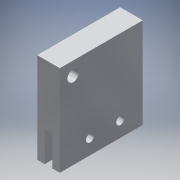
# Autodesk Inventor part: NarrowSupportForLift
Saved by Autodesk Inventor 2016 SP1 (Build 200210100, 210)
## iProperties
Created: 2016-02-14
Part Number: NarrowSupportForLift
Material: Aluminum 6061
Document SubType Name: Modeling
Designer: steele
Density: 2.7 g/cm^3
Appearance: Aluminum - Flat
Mass: 237.224 g
Surface Area: 201.153 cm^2
Volume: 87.8608 cm^3
Author: steele
Autodesk Inventor part; units mm, degrees
ref_plane "YZ Plane" through (0, 0, 0) normal (1, 0, 0) x (0, 1, 0)
ref_plane "XZ Plane" through (0, 0, 0) normal (0, 1, 0) x (-1, 0, 0)
ref_plane "XY Plane" through (0, 0, 0) normal (0, 0, 1) x (1, 0, 0)
sketch "Sketch4" plane through (0, 0, 0) normal (1, 0, 0) x (0, 1, 0)
  line L0 (-25.4, 34.925) -> (-25.4, -34.925)
  line L1 (-25.4, -34.925) -> (0, -34.925)
  line L2 (0, -34.925) -> (0, 34.925)
  line L3 (0, 34.925) -> (-25.4, 34.925)
  line L4 (-25.4, -34.925) -> (-12.7, 0) construction
  line L5 (0, 34.925) -> (50.8, 34.925)
  line L6 (50.8, 34.925) -> (50.8, -34.925)
  line L7 (50.8, -34.925) -> (0, -34.925)
  line L8 (0, -34.925) -> (0, 34.925)
  circle A0 centre (39.6875, 23.8125) radius 4.7625
  circle A1 centre (39.6875, -23.8125) radius 4.7625
  point P0 (0, 0)
  point P1 (-12.7, 0)
  dimension "d2" = 69.85
  dimension "d3" = 25.4
  dimension "d12" = 50.8
  dimension "d15" = 9.525
  dimension "d16" = 11.1125
  dimension "d23" = 11.1125
  dimension "d26" = 11.1125
  constraints: 18 end point, 4 parallel, 2 centre point, 2 perpendicular, 1 collinear, 1 equal radius, 1 horizontal, 1 point on line, 1 vertical
  measures "d2" distance of L0.start L0.end
  measures "d3" distance of L2.end L0.start
  measures "d12" distance of L2.end L5.end
  measures "d15" diameter of A0
  measures "d16" distance from line of A0.centre L6
  measures "d23" distance from line of A0.centre L5
  measures "d26" distance from line of A1.centre L7
extrude "Extrusion3" add sketch "Sketch4" along normal mid plane 19.05 contours L3 L2 L1 L0 | L5 L6 L7 L2 | A1
sketch "Sketch6" plane through (-9.525, -25.4, 34.925) normal (0, 0, 1) x (1, 0, 0)
  line L0 (9.525, 25.4) -> (9.525, 0) construction
  line L1 (0, 0) -> (19.05, 0) construction
  line L2 (6.35, 0) -> (12.7, 0)
  line L3 (12.7, 0) -> (12.7, 25.4)
  line L4 (12.7, 25.4) -> (6.35, 25.4)
  line L5 (6.35, 25.4) -> (6.35, 0)
  line L6 (6.35, 0) -> (12.7, 25.4) construction
  line L7 (12.7, 0) -> (6.35, 25.4) construction
  point P0 (9.525, 12.7)
  dimension "d20" = 6.35
  constraints: 14 end point, 4 midpoint, 2 parallel, 1 horizontal, 1 perpendicular
  measures "d20" distance between parallel lines of L3 L5
extrude "Extrusion4" cut sketch "Sketch6" against normal through all
sketch "Sketch7" plane through (9.525, 0, 0) normal (1, 0, 0) x (0, 0, -1)
  line L0 (34.925, -25.4) -> (34.925, 0) projected
  line L1 (-34.925, -25.4) -> (34.925, -25.4) projected
  line L2 (-34.925, 0) -> (-34.925, -25.4) projected
  line L3 (-34.925, 0) -> (34.925, 0) projected
  line L4 (-34.925, -85.725) -> (-34.925, -12.7) projected
  arc A0 (-34.925, -85.725) -> (-22.225, -98.425) centre (-22.225, -85.725) ccw projected
  line L5 (479.425, -98.425) -> (-22.225, -98.425) projected
  arc A1 (479.425, -98.425) -> (492.125, -85.725) centre (479.425, -85.725) ccw projected
  line L6 (492.125, -81.1401) -> (492.125, -85.725) projected
  arc A2 (492.125, -81.1401) -> (488.7869, -72.5584) centre (479.425, -81.1401) ccw projected
  line L7 (488.7869, -72.5584) -> (426.0501, -4.1183) projected
  arc A3 (426.0501, -4.1183) -> (416.6882, 0) centre (416.6882, -12.7) ccw projected
  line L8 (416.6882, 0) -> (-22.225, 0) projected
  arc A4 (-22.225, 0) -> (-34.925, -12.7) centre (-22.225, -12.7) ccw projected
  circle A5 centre (473.075, -79.375) radius 4.826 projected
  circle A6 centre (15.875, -79.375) radius 4.826 projected
  circle A7 centre (457.2, -79.375) radius 4.826 projected
  circle A8 centre (440.1745, -40.6685) radius 3.3782 projected
  circle A9 centre (422.275, -85.725) radius 3.3782 projected
  line L9 (20.6375, -55.8157) -> (20.6375, -25.4) projected
  arc A10 (23.8125, -22.225) -> (20.6375, -25.4) centre (23.8125, -25.4) ccw projected
  line L10 (23.8125, -22.225) -> (46.9319, -22.225) projected
  arc A11 (49.4596, -27.3213) -> (46.9319, -22.225) centre (46.9319, -25.4) ccw projected
  line L11 (49.4596, -27.3213) -> (26.3402, -57.737) projected
  arc A12 (20.6375, -55.8157) -> (26.3402, -57.737) centre (23.8125, -55.8157) ccw projected
  line L12 (28.1443, -71.1037) -> (56.0904, -34.338) projected
  arc A13 (61.7931, -36.2593) -> (56.0904, -34.338) centre (58.6181, -36.2593) ccw projected
  line L13 (61.7931, -36.2593) -> (61.7931, -73.025) projected
  arc A14 (58.6181, -76.2) -> (61.7931, -73.025) centre (58.6181, -73.025) ccw projected
  line L14 (58.6181, -76.2) -> (30.672, -76.2) projected
  arc A15 (28.1443, -71.1037) -> (30.672, -76.2) centre (30.672, -73.025) ccw projected
  line L15 (184.056, -73.025) -> (184.056, -34.8804) projected
  arc A16 (189.5742, -32.738) -> (184.056, -34.8804) centre (187.231, -34.8804) ccw projected
  line L16 (189.5742, -32.738) -> (224.451, -70.8826) projected
  arc A17 (222.1078, -76.2) -> (224.451, -70.8826) centre (222.1078, -73.025) ccw projected
  line L17 (222.1078, -76.2) -> (187.231, -76.2) projected
  arc A18 (184.056, -73.025) -> (187.231, -76.2) centre (187.231, -73.025) ccw projected
  line L18 (291.2199, -27.5424) -> (254.7557, -67.4233) projected
  arc A19 (249.2375, -65.2808) -> (254.7557, -67.4233) centre (252.4125, -65.2808) ccw projected
  line L19 (249.2375, -65.2808) -> (249.2375, -25.4) projected
  arc A20 (252.4125, -22.225) -> (249.2375, -25.4) centre (252.4125, -25.4) ccw projected
  line L20 (252.4125, -22.225) -> (288.8767, -22.225) projected
  arc A21 (291.2199, -27.5424) -> (288.8767, -22.225) centre (288.8767, -25.4) ccw projected
  line L21 (234.1943, -67.4233) -> (197.7301, -27.5424) projected
  arc A22 (200.0733, -22.225) -> (197.7301, -27.5424) centre (200.0733, -25.4) ccw projected
  line L22 (200.0733, -22.225) -> (236.5375, -22.225) projected
  arc A23 (239.7125, -25.4) -> (236.5375, -22.225) centre (236.5375, -25.4) ccw projected
  line L23 (239.7125, -25.4) -> (239.7125, -65.2808) projected
  arc A24 (234.1943, -67.4233) -> (239.7125, -65.2808) centre (236.5375, -65.2808) ccw projected
  line L24 (304.894, -34.8804) -> (304.894, -73.025) projected
  arc A25 (301.719, -76.2) -> (304.894, -73.025) centre (301.719, -73.025) ccw projected
  line L25 (301.719, -76.2) -> (266.8422, -76.2) projected
  arc A26 (264.499, -70.8826) -> (266.8422, -76.2) centre (266.8422, -73.025) ccw projected
  line L26 (264.499, -70.8826) -> (299.3758, -32.738) projected
  arc A27 (304.894, -34.8804) -> (299.3758, -32.738) centre (301.719, -34.8804) ccw projected
  line L27 (341.3125, -25.4) -> (341.3125, -73.025) projected
  arc A28 (338.1375, -76.2) -> (341.3125, -73.025) centre (338.1375, -73.025) ccw projected
  line L28 (338.1375, -76.2) -> (317.594, -76.2) projected
  arc A29 (314.419, -73.025) -> (317.594, -76.2) centre (317.594, -73.025) ccw projected
  line L29 (314.419, -73.025) -> (314.419, -25.4) projected
  arc A30 (317.594, -22.225) -> (314.419, -25.4) centre (317.594, -25.4) ccw projected
  line L30 (317.594, -22.225) -> (338.1375, -22.225) projected
  arc A31 (341.3125, -25.4) -> (338.1375, -22.225) centre (338.1375, -25.4) ccw projected
  line L31 (400.05, -69.85) -> (400.05, -29.1831) projected
  arc A32 (405.5794, -27.053) -> (400.05, -29.1831) centre (403.225, -29.1831) ccw projected
  line L32 (405.5794, -27.053) -> (445.2458, -70.8949) projected
  arc A33 (442.8915, -76.2) -> (445.2458, -70.8949) centre (442.8915, -73.025) ccw projected
  line L33 (442.8915, -76.2) -> (406.4, -76.2) projected
  arc A34 (400.05, -69.85) -> (406.4, -76.2) centre (406.4, -69.85) ccw projected
  circle A35 centre (83.3958, -57.6072) radius 5.5626 projected
  circle A36 centre (160.8658, -32.2072) radius 5.5626 projected
  circle A37 centre (83.3958, -32.2072) radius 5.5626 projected
  circle A38 centre (160.8658, -57.6072) radius 5.5626 projected
  circle A39 centre (358.775, -28.575) radius 2.5527 projected
  circle A40 centre (368.3, -19.05) radius 2.5527 projected
  circle A41 centre (377.825, -9.525) radius 2.5527 projected
  circle A42 centre (358.775, -88.9) radius 2.5527 projected
  circle A43 centre (377.825, -69.85) radius 2.5527 projected
  circle A44 centre (368.3, -79.375) radius 2.5527 projected
  circle A45 centre (-9.525, -12.7) radius 3.3782 projected
  circle A46 centre (-9.525, -85.725) radius 3.3782 projected
  circle A47 centre (15.875, -12.7) radius 3.3782 projected
  circle A48 centre (41.275, -12.7) radius 3.3782 projected
  circle A49 centre (41.275, -85.725) radius 3.3782 projected
  circle A50 centre (66.675, -12.7) radius 3.3782 projected
  circle A51 centre (92.075, -12.7) radius 3.3782 projected
  circle A52 centre (92.075, -85.725) radius 3.3782 projected
  circle A53 centre (117.475, -12.7) radius 3.3782 projected
  circle A54 centre (117.475, -85.725) radius 3.3782 projected
  circle A55 centre (142.875, -12.7) radius 3.3782 projected
  circle A56 centre (142.875, -85.725) radius 3.3782 projected
  circle A57 centre (168.275, -12.7) radius 3.3782 projected
  circle A58 centre (193.675, -12.7) radius 3.3782 projected
  circle A59 centre (193.675, -85.725) radius 3.3782 projected
  circle A60 centre (219.075, -12.7) radius 3.3782 projected
  circle A61 centre (219.075, -85.725) radius 3.3782 projected
  circle A62 centre (244.475, -12.7) radius 3.3782 projected
  circle A63 centre (269.875, -12.7) radius 3.3782 projected
  circle A64 centre (269.875, -85.725) radius 3.3782 projected
  circle A65 centre (295.275, -12.7) radius 3.3782 projected
  circle A66 centre (295.275, -85.725) radius 3.3782 projected
  circle A67 centre (320.675, -12.7) radius 3.3782 projected
  circle A68 centre (320.675, -85.725) radius 3.3782 projected
  circle A69 centre (346.075, -12.7) radius 3.3782 projected
  circle A70 centre (346.075, -85.725) radius 3.3782 projected
  circle A71 centre (396.875, -12.7) radius 3.3782 projected
  circle A72 centre (396.875, -85.725) radius 3.3782 projected
  circle A73 centre (419.1, -15.875) radius 4.953 projected
  circle A74 centre (66.5556, -90.5002) radius 3.3528 projected
  circle A75 centre (177.706, -90.5002) radius 3.3528 projected
  circle A76 centre (122.1308, -60.325) radius 14.2812 projected
  circle A77 centre (244.475, -83.185) radius 4.826 projected
  circle A78 centre (-9.525, -12.7) radius 3.3782
  circle A79 centre (15.875, -12.7) radius 3.3782
  point P0 (0, 0)
  constraints: 2 centre point, 2 coincident, 2 concentric
extrude "Extrusion5" cut sketch "Sketch7" against normal through all contours A45 | A47
sketch "Sketch8" plane through (9.525, 0, 0) normal (1, 0, 0) x (0, 0, -1)
  circle A0 centre (-23.8125, 39.6875) radius 4.7625 projected
  circle A1 centre (23.8125, 39.6875) radius 4.7625
  line L0 (34.925, -25.4) -> (34.925, 50.8) projected
  point P0 (0, 0)
  dimension "d27" = 11.1125
  constraints: 1 centre point, 1 equal radius
  measures "d27" distance from line of A1.centre L0
extrude "Extrusion6" cut sketch "Sketch8" against normal through all contours A1
body "Solid2"
